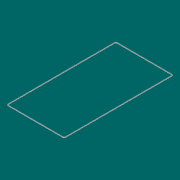
# Autodesk Inventor part: topORing
Saved by Autodesk Inventor 2016 SP1 (Build 200210100, 210)
## iProperties
Created: 2015-10-27
Part Number: topORing
Material: Rubber
Document SubType Name: Modeling
Designer: Sawaiz
Density: 0.93 g/cm^3
Appearance: Rubber - Black
Author: Sawaiz
Autodesk Inventor part; units mm, degrees
ref_plane "YZ Plane" through (0, 0, 0) normal (1, 0, 0) x (0, 1, 0)
ref_plane "XZ Plane" through (0, 0, 0) normal (0, 1, 0) x (-1, 0, 0)
ref_plane "XY Plane" through (0, 0, 0) normal (0, 0, 1) x (1, 0, 0)
sketch "Sketch1" plane through (0, 0, 0) normal (0, 0, 1) x (1, 0, 0)
  line L0 (146.05, -73.025) -> (-146.05, -73.025)
  line L1 (-146.05, -73.025) -> (-146.05, 73.025)
  line L2 (-146.05, 73.025) -> (146.05, 73.025)
  line L3 (146.05, 73.025) -> (146.05, -73.025)
  line L4 (146.05, -73.025) -> (-146.05, 73.025) construction
  line L5 (-146.05, -73.025) -> (146.05, 73.025) construction
  line L6 (-144.4625, 67.0179) -> (-144.4625, -67.0179)
  line L7 (-140.0429, -71.4375) -> (140.0429, -71.4375)
  line L8 (144.4625, -67.0179) -> (144.4625, 67.0179)
  line L9 (140.0429, 71.4375) -> (-140.0429, 71.4375)
  line L10 (-142.2527, -67.0179) -> (-142.2527, 67.0179)
  line L11 (-140.0429, 69.2277) -> (140.0429, 69.2277)
  line L12 (142.2527, 67.0179) -> (142.2527, -67.0179)
  line L13 (140.0429, -69.2277) -> (-140.0429, -69.2277)
  arc A0 (-142.2527, -67.0179) -> (-140.0429, -69.2277) centre (-140.0429, -67.0179) ccw
  arc A1 (140.0429, -69.2277) -> (142.2527, -67.0179) centre (140.0429, -67.0179) ccw
  arc A2 (142.2527, 67.0179) -> (140.0429, 69.2277) centre (140.0429, 67.0179) ccw
  arc A3 (-140.0429, 69.2277) -> (-142.2527, 67.0179) centre (-140.0429, 67.0179) ccw
  arc A4 (-144.4625, -67.0179) -> (-140.0429, -71.4375) centre (-140.0429, -67.0179) ccw
  arc A5 (140.0429, -71.4375) -> (144.4625, -67.0179) centre (140.0429, -67.0179) ccw
  arc A6 (144.4625, 67.0179) -> (140.0429, 71.4375) centre (140.0429, 67.0179) ccw
  arc A7 (-140.0429, 71.4375) -> (-144.4625, 67.0179) centre (-140.0429, 67.0179) ccw
  point P0 (0, 0)
  dimension "d0" = 292.1
  dimension "d1" = 146.05
  dimension "d2" = 1.5875
  dimension "d3" = 2.2098
  dimension "d4" = 2.2098
  dimension "d5" = 4.4196
  constraints: 28 end point, 16 point on circle, 16 tangent, 8 centre point, 6 equal radius, 6 parallel, 3 perpendicular, 2 midpoint, 1 horizontal, 6 other
  measures "d0" distance of L1.end L2.end
  measures "d1" distance of L0.end L1.end
  measures "d2" distance between parallel lines of L1 L6
  measures "d3" distance between parallel lines of L6 L10
  measures "d4" radius of A0
  measures "d5" radius of A4
extrude "Extrusion1" add sketch "Sketch1" along normal blind 1.1684 contours A7 L9 A6 L8 A5 L7 A4 L6
fillet "Fillet1" radius 0.5 32 edges at (-141.6055, 68.5805, 1.1684) (0, 69.2277, 1.1684) (141.6055, 68.5805, 1.1684) (142.2527, 0, 1.1684) (141.6055, -68.5805, 1.1684) (0, -69.2277, 1.1684) (-141.6055, -68.5805, 1.1684) (-142.2527, 0, 1.1684) (-141.6055, 68.5805, 0) (-142.2527, 0, 0) (-141.6055, -68.5805, 0) (0, -69.2277, 0) (141.6055, -68.5805, 0) (142.2527, 0, 0) (141.6055, 68.5805, 0) (0, 69.2277, 0) (-144.4625, 0, 1.1684) (-143.168, -70.143, 1.1684) (0, -71.4375, 1.1684) (143.168, -70.143, 1.1684) (144.4625, 0, 1.1684) (143.168, 70.143, 1.1684) (0, 71.4375, 1.1684) (-143.168, 70.143, 1.1684) (-144.4625, 0, 0) (-143.168, 70.143, 0) (0, 71.4375, 0) (143.168, 70.143, 0) (144.4625, 0, 0) (143.168, -70.143, 0) (0, -71.4375, 0) (-143.168, -70.143, 0)
equation "\"d0\" = depth + 2 * frameAcrylicThickness"
equation "\"d1\" = width + 2 * frameAcrylicThickness"
equation "\"frameAcrylicThickness\" = 9.525"
equation "\"width\" = 127"
equation "\"depth\" = 273.05"
equation "\"internalAcrylicThickness\" = 6.35"
equation "\"height\" = 127"
equation "\"mirrorAngle\" = 5deg"
equation "\"detectorWidth\" = 52"
equation "\"detectorHeight\" = 52"
equation "\"mirrorThickness\" = 3.175"
equation "\"fresnelThickness\" = 0.1"
equation "\"focalLength\" = 76.2"
equation "\"ior\" = 1.49"
equation "\"centerThickness\" = 1.524"
equation "\"fresnelAngle\" = 90deg"
equation "\"fresnelEffectiveDiameter\" = 152.4"
equation "\"oRingWidth\" = 1.5875"
equation "\"sensorHolderDepth\" = 19.05"
equation "\"aerogelClearence\" = 3.175"
equation "\"backplanePCBHeight\" = 76.2"
equation "\"backplanePCBWidth\" = 76.2"
equation "\"backplaneHoleOffsett\" = 6.35"
equation "\"backplanePostionOffsett\" = 12.7"
equation "\"moduleSlotClearence\" = 0.79375"
body "Solid1"
